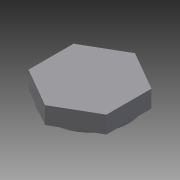
# Autodesk Inventor part: 13_8
Saved by Autodesk Inventor 2015 (Build 190159000, 159)
## iProperties
Created: 2015-04-01
Part Number: 13_8
Material: Generic
Document SubType Name: Modeling
Designer: WASHHSST
Density: 1 g/cm^3
Appearance: Default
Author: WASHHSST
Autodesk Inventor part; units mm, degrees
ref_plane "YZ Plane" through (0, 0, 0) normal (1, 0, 0) x (0, 1, 0)
ref_plane "XZ Plane" through (0, 0, 0) normal (0, 1, 0) x (-1, 0, 0)
ref_plane "XY Plane" through (0, 0, 0) normal (0, 0, 1) x (1, 0, 0)
sketch "Sketch1" plane through (0, 0, 0) normal (0, 1, 0) x (-1, 0, 0)
  circle A0 centre (0, 0) radius 9.9187
  line L0 (9.9187, -5.7266) -> (0, -11.4531)
  line L1 (0, -11.4531) -> (-9.9187, -5.7266)
  line L2 (-9.9187, -5.7266) -> (-9.9187, 5.7266)
  line L3 (-9.9187, 5.7266) -> (0, 11.4531)
  line L4 (0, 11.4531) -> (9.9187, 5.7266)
  line L5 (9.9187, 5.7266) -> (9.9187, -5.7266)
  line L6 (0, 13.376) -> (0, -12.9473) construction
  point P0 (9.9187, 0)
  dimension "d0" = 19.8374
  constraints: 14 end point, 2 coincident, 1 horizontal alignment, 1 midpoint, 1 parallel, 1 vertical, 15 other
extrude "Extrusion1" add sketch "Sketch1" along normal blind 4.3688
sketch "Sketch2" plane through (0, 0, 0) normal (0, -1, 0) x (1, 0, 0)
  circle A0 centre (0, 0) radius 9.9187
  line L0 (0, 11.4531) -> (9.9187, 5.7266) projected
  constraints: 1 centre point, 1 coincident, 1 tangent
extrude "Extrusion2" add sketch "Sketch2" along normal blind 0.4064
body "Solid1"
